Autodesk Fusion 360 part; units mm, degrees
(part 5 of 7)
  spline S10 degree 5 poles (-24.1252, -41.4832) (-24.1281, -41.4894) (-24.1337, -41.5019) (-24.1416, -41.5208) (-24.1514, -41.5463) (-24.1624, -41.5787) (-24.1725, -41.6115) (-24.1821, -41.6445) (-24.1913, -41.6776) (-24.2004, -41.7108) (-24.2093, -41.7442) (-24.2179, -41.7776) (-24.2261, -41.8112) (-24.2339, -41.8449) (-24.2413, -41.8788) (-24.2483, -41.9128) (-24.255, -41.947) (-24.2613, -41.9813) (-24.2675, -42.0157) (-24.2734, -42.0502) (-24.279, -42.0847) (-24.2844, -42.1193) (-24.2896, -42.1541) (-24.2944, -42.1889) (-24.299, -42.2238) (-24.3034, -42.2588) (-24.3075, -42.2939) (-24.3114, -42.3291) (-24.315, -42.3643) (-24.3185, -42.3996) (-24.3217, -42.435) (-24.3247, -42.4705) (-24.3275, -42.506) (-24.33, -42.5416) (-24.3324, -42.5773) (-24.3345, -42.613) (-24.3364, -42.6488) (-24.3382, -42.6847) (-24.3397, -42.7206) (-24.341, -42.7565) (-24.3421, -42.7926) (-24.343, -42.8287) (-24.3438, -42.8648) (-24.3443, -42.901) (-24.3446, -42.9372) (-24.3448, -42.9735) (-24.3447, -43.0099) (-24.3445, -43.0463) (-24.3441, -43.0828) (-24.3435, -43.1193) (-24.3427, -43.1558) (-24.3418, -43.1924) (-24.3406, -43.229) (-24.3393, -43.2657) (-24.3378, -43.3024) (-24.3361, -43.3392) (-24.3342, -43.376) (-24.3322, -43.4129) (-24.33, -43.4497) (-24.3276, -43.4867) (-24.325, -43.5236) (-24.3223, -43.5606) (-24.3194, -43.5977) (-24.3163, -43.6348) (-24.3131, -43.6719) (-24.3097, -43.709) (-24.3061, -43.7462) (-24.3024, -43.7834) (-24.2985, -43.8206) (-24.2944, -43.8579) (-24.2901, -43.8952) (-24.2866, -43.9251) (-24.2839, -43.9475) (-24.2821, -43.9625) (-24.2811, -43.9699) knots 0 0 0 0 0 0 0.01428571 0.02857143 0.04285714 0.05714286 0.07142857 0.08571429 0.1 0.11428571 0.12857143 0.14285714 0.15714286 0.17142857 0.18571429 0.2 0.21428571 0.22857143 0.24285714 0.25714286 0.27142857 0.28571429 0.3 0.31428571 0.32857143 0.34285714 0.35714286 0.37142857 0.38571429 0.4 0.41428571 0.42857143 0.44285714 0.45714286 0.47142857 0.48571429 0.5 0.51428571 0.52857143 0.54285714 0.55714286 0.57142857 0.58571429 0.6 0.61428571 0.62857143 0.64285714 0.65714286 0.67142857 0.68571429 0.7 0.71428571 0.72857143 0.74285714 0.75714286 0.77142857 0.78571429 0.8 0.81428571 0.82857143 0.84285714 0.85714286 0.87142857 0.88571429 0.9 0.91428571 0.92857143 0.94285714 0.95714286 0.97142857 0.98571429 1 1 1 1 1 1
  arc A22 (-24.2811, -43.9699) -> (-23.453, -44.284) centre (-17.3506, -26.9445) ccw
  spline S11 degree 5 poles (-23.453, -44.284) (-23.4474, -44.279) (-23.4361, -44.2691) (-23.4192, -44.2541) (-23.3967, -44.2341) (-23.3688, -44.2089) (-23.341, -44.1837) (-23.3134, -44.1585) (-23.2859, -44.1331) (-23.2586, -44.1076) (-23.2314, -44.0821) (-23.2044, -44.0565) (-23.1775, -44.0307) (-23.1508, -44.0049) (-23.1242, -43.9791) (-23.0978, -43.9531) (-23.0715, -43.927) (-23.0454, -43.9009) (-23.0194, -43.8747) (-22.9936, -43.8483) (-22.968, -43.8219) (-22.9425, -43.7954) (-22.9172, -43.7689) (-22.892, -43.7422) (-22.867, -43.7155) (-22.8422, -43.6886) (-22.8176, -43.6617) (-22.7931, -43.6347) (-22.7688, -43.6076) (-22.7446, -43.5804) (-22.7207, -43.5531) (-22.6969, -43.5258) (-22.6733, -43.4983) (-22.6499, -43.4708) (-22.6266, -43.4432) (-22.6036, -43.4155) (-22.5807, -43.3877) (-22.558, -43.3598) (-22.5355, -43.3318) (-22.5132, -43.3037) (-22.4912, -43.2756) (-22.4693, -43.2473) (-22.4476, -43.219) (-22.4261, -43.1905) (-22.4048, -43.162) (-22.3838, -43.1334) (-22.3629, -43.1047) (-22.3423, -43.0759) (-22.3219, -43.047) (-22.3017, -43.018) (-22.2817, -42.9889) (-22.262, -42.9597) (-22.2426, -42.9304) (-22.2234, -42.901) (-22.2045, -42.8715) (-22.1858, -42.8419) (-22.1673, -42.8122) (-22.1491, -42.7824) (-22.1312, -42.7525) (-22.1135, -42.7225) (-22.0961, -42.6924) (-22.0792, -42.6621) (-22.0627, -42.6316) (-22.0466, -42.6011) (-22.0308, -42.5703) (-22.0154, -42.5395) (-22.0001, -42.5086) (-21.9851, -42.4777) (-21.9704, -42.4466) (-21.9562, -42.4154) (-21.943, -42.3838) (-21.9333, -42.3583) (-21.9267, -42.3389) (-21.9227, -42.3258) (-21.9207, -42.3193) knots -1 -1 -1 -1 -1 -1 -0.98571429 -0.97142857 -0.95714286 -0.94285714 -0.92857143 -0.91428571 -0.9 -0.88571429 -0.87142857 -0.85714286 -0.84285714 -0.82857143 -0.81428571 -0.8 -0.78571429 -0.77142857 -0.75714286 -0.74285714 -0.72857143 -0.71428571 -0.7 -0.68571429 -0.67142857 -0.65714286 -0.64285714 -0.62857143 -0.61428571 -0.6 -0.58571429 -0.57142857 -0.55714286 -0.54285714 -0.52857143 -0.51428571 -0.5 -0.48571429 -0.47142857 -0.45714286 -0.44285714 -0.42857143 -0.41428571 -0.4 -0.38571429 -0.37142857 -0.35714286 -0.34285714 -0.32857143 -0.31428571 -0.3 -0.28571429 -0.27142857 -0.25714286 -0.24285714 -0.22857143 -0.21428571 -0.2 -0.18571429 -0.17142857 -0.15714286 -0.14285714 -0.12857143 -0.11428571 -0.1 -0.08571429 -0.07142857 -0.05714286 -0.04285714 -0.02857143 -0.01428571 0 0 0 0 0 0
  line L11 (-21.9207, -42.3193) -> (-21.8906, -42.2182)
  arc A23 (-21.2841, -41.8777) -> (-21.8906, -42.2182) centre (-21.4115, -42.3612) ccw
  arc A24 (-21.2841, -41.8777) -> (-20.8075, -41.9952) centre (-17.3506, -26.9445) ccw
  arc A25 (-20.4288, -42.5785) -> (-20.8075, -41.9952) centre (-20.9195, -42.4825) ccw
  line L12 (-20.4288, -42.5785) -> (-20.449, -42.682)
  spline S12 degree 5 poles (-20.449, -42.682) (-20.4503, -42.6887) (-20.4528, -42.7022) (-20.456, -42.7224) (-20.4593, -42.7495) (-20.4622, -42.7836) (-20.4642, -42.8179) (-20.4656, -42.8522) (-20.4667, -42.8866) (-20.4675, -42.921) (-20.4682, -42.9555) (-20.4685, -42.99) (-20.4685, -43.0246) (-20.468, -43.0592) (-20.4671, -43.0939) (-20.4657, -43.1286) (-20.464, -43.1634) (-20.462, -43.1982) (-20.4597, -43.2331) (-20.4572, -43.2679) (-20.4544, -43.3028) (-20.4513, -43.3378) (-20.448, -43.3727) (-20.4444, -43.4077) (-20.4406, -43.4427) (-20.4364, -43.4777) (-20.432, -43.5128) (-20.4273, -43.5479) (-20.4225, -43.583) (-20.4173, -43.6181) (-20.412, -43.6532) (-20.4064, -43.6883) (-20.4006, -43.7235) (-20.3946, -43.7587) (-20.3883, -43.7939) (-20.3819, -43.8291) (-20.3752, -43.8643) (-20.3682, -43.8995) (-20.3611, -43.9347) (-20.3538, -43.97) (-20.3463, -44.0052) (-20.3385, -44.0405) (-20.3306, -44.0758) (-20.3224, -44.111) (-20.3141, -44.1463) (-20.3055, -44.1816) (-20.2968, -44.2169) (-20.2879, -44.2522) (-20.2787, -44.2875) (-20.2694, -44.3228) (-20.2599, -44.358) (-20.2502, -44.3933) (-20.2404, -44.4286) (-20.2303, -44.4639) (-20.22, -44.4992) (-20.2096, -44.5345) (-20.199, -44.5698) (-20.1882, -44.6051) (-20.1772, -44.6404) (-20.1661, -44.6757) (-20.1547, -44.711) (-20.1432, -44.7462) (-20.1315, -44.7815) (-20.1197, -44.8168) (-20.1077, -44.852) (-20.0955, -44.8873) (-20.0831, -44.9225) (-20.0705, -44.9578) (-20.0578, -44.993) (-20.045, -45.0282) (-20.0319, -45.0634) (-20.0213, -45.0916) (-20.0133, -45.1127) (-20.008, -45.1268) (-20.0053, -45.1338) knots 0 0 0 0 0 0 0.01428571 0.02857143 0.04285714 0.05714286 0.07142857 0.08571429 0.1 0.11428571 0.12857143 0.14285714 0.15714286 0.17142857 0.18571429 0.2 0.21428571 0.22857143 0.24285714 0.25714286 0.27142857 0.28571429 0.3 0.31428571 0.32857143 0.34285714 0.35714286 0.37142857 0.38571429 0.4 0.41428571 0.42857143 0.44285714 0.45714286 0.47142857 0.48571429 0.5 0.51428571 0.52857143 0.54285714 0.55714286 0.57142857 0.58571429 0.6 0.61428571 0.62857143 0.64285714 0.65714286 0.67142857 0.68571429 0.7 0.71428571 0.72857143 0.74285714 0.75714286 0.77142857 0.78571429 0.8 0.81428571 0.82857143 0.84285714 0.85714286 0.87142857 0.88571429 0.9 0.91428571 0.92857143 0.94285714 0.95714286 0.97142857 0.98571429 1 1 1 1 1 1
  arc A26 (-20.0053, -45.1338) -> (-19.1261, -45.2405) centre (-17.3506, -26.9445) ccw
  spline S13 degree 5 poles (-19.1261, -45.2405) (-19.1218, -45.2344) (-19.1132, -45.222) (-19.1004, -45.2034) (-19.0834, -45.1786) (-19.0623, -45.1475) (-19.0414, -45.1164) (-19.0206, -45.0852) (-19, -45.054) (-18.9795, -45.0228) (-18.9592, -44.9915) (-18.9391, -44.9601) (-18.9192, -44.9287) (-18.8994, -44.8973) (-18.8798, -44.8658) (-18.8603, -44.8342) (-18.8411, -44.8026) (-18.822, -44.771) (-18.803, -44.7393) (-18.7843, -44.7076) (-18.7657, -44.6758) (-18.7473, -44.644) (-18.7291, -44.6121) (-18.711, -44.5802) (-18.6932, -44.5483) (-18.6755, -44.5163) (-18.658, -44.4843) (-18.6407, -44.4522) (-18.6236, -44.42) (-18.6067, -44.3879) (-18.5899, -44.3557) (-18.5734, -44.3234) (-18.557, -44.2911) (-18.5409, -44.2588) (-18.5249, -44.2264) (-18.5092, -44.194) (-18.4936, -44.1615) (-18.4783, -44.129) (-18.4631, -44.0964) (-18.4482, -44.0639) (-18.4335, -44.0312) (-18.419, -43.9986) (-18.4047, -43.9658) (-18.3907, -43.9331) (-18.3769, -43.9003) (-18.3633, -43.8675) (-18.3499, -43.8346) (-18.3367, -43.8017) (-18.3238, -43.7688) (-18.3112, -43.7358) (-18.2988, -43.7028) (-18.2866, -43.6697) (-18.2747, -43.6366) (-18.2632, -43.6034) (-18.2518, -43.5703) (-18.2408, -43.537) (-18.23, -43.5038) (-18.2194, -43.4705) (-18.2091, -43.4372) (-18.1992, -43.4038) (-18.1895, -43.3704) (-18.1803, -43.337) (-18.1716, -43.3035) (-18.1633, -43.2699) (-18.1553, -43.2363) (-18.1477, -43.2027) (-18.1403, -43.1691) (-18.1331, -43.1354) (-18.1262, -43.1017) (-18.12, -43.068) (-18.1146, -43.0342) (-18.1114, -43.0071) (-18.1097, -42.9867) (-18.1088, -42.973) (-18.1085, -42.9662) knots -1 -1 -1 -1 -1 -1 -0.98571429 -0.97142857 -0.95714286 -0.94285714 -0.92857143 -0.91428571 -0.9 -0.88571429 -0.87142857 -0.85714286 -0.84285714 -0.82857143 -0.81428571 -0.8 -0.78571429 -0.77142857 -0.75714286 -0.74285714 -0.72857143 -0.71428571 -0.7 -0.68571429 -0.67142857 -0.65714286 -0.64285714 -0.62857143 -0.61428571 -0.6 -0.58571429 -0.57142857 -0.55714286 -0.54285714 -0.52857143 -0.51428571 -0.5 -0.48571429 -0.47142857 -0.45714286 -0.44285714 -0.42857143 -0.41428571 -0.4 -0.38571429 -0.37142857 -0.35714286 -0.34285714 -0.32857143 -0.31428571 -0.3 -0.28571429 -0.27142857 -0.25714286 -0.24285714 -0.22857143 -0.21428571 -0.2 -0.18571429 -0.17142857 -0.15714286 -0.14285714 -0.12857143 -0.11428571 -0.1 -0.08571429 -0.07142857 -0.05714286 -0.04285714 -0.02857143 -0.01428571 0 0 0 0 0 0
  line L13 (-18.1085, -42.9662) -> (-18.1034, -42.8608)
  arc A27 (-17.596, -42.3851) -> (-18.1034, -42.8608) centre (-17.604, -42.8851) ccw
  arc A28 (-17.596, -42.3851) -> (-17.1052, -42.3851) centre (-17.3506, -26.9445) ccw
  arc A29 (-16.5978, -42.8608) -> (-17.1052, -42.3851) centre (-17.0973, -42.8851) ccw
  line L14 (-16.5978, -42.8608) -> (-16.5927, -42.9662)
  spline S14 degree 5 poles (-16.5927, -42.9662) (-16.5924, -42.973) (-16.5916, -42.9867) (-16.5898, -43.0071) (-16.5866, -43.0342) (-16.5813, -43.068) (-16.575, -43.1017) (-16.5681, -43.1354) (-16.5609, -43.1691) (-16.5535, -43.2027) (-16.5459, -43.2363) (-16.538, -43.2699) (-16.5297, -43.3035) (-16.5209, -43.337) (-16.5117, -43.3704) (-16.5021, -43.4038) (-16.4921, -43.4372) (-16.4818, -43.4705) (-16.4712, -43.5038) (-16.4604, -43.537) (-16.4494, -43.5703) (-16.4381, -43.6034) (-16.4265, -43.6366) (-16.4146, -43.6697) (-16.4025, -43.7028) (-16.3901, -43.7358) (-16.3774, -43.7688) (-16.3645, -43.8017) (-16.3513, -43.8346) (-16.338, -43.8675) (-16.3244, -43.9003) (-16.3106, -43.9331) (-16.2965, -43.9658) (-16.2822, -43.9986) (-16.2677, -44.0312) (-16.253, -44.0639) (-16.2381, -44.0964) (-16.223, -44.129) (-16.2076, -44.1615) (-16.1921, -44.194) (-16.1763, -44.2264) (-16.1604, -44.2588) (-16.1442, -44.2911) (-16.1279, -44.3234) (-16.1113, -44.3557) (-16.0946, -44.3879) (-16.0776, -44.42) (-16.0605, -44.4522) (-16.0432, -44.4843) (-16.0257, -44.5163) (-16.008, -44.5483) (-15.9902, -44.5802) (-15.9721, -44.6121) (-15.9539, -44.644) (-15.9355, -44.6758) (-15.9169, -44.7076) (-15.8982, -44.7393) (-15.8793, -44.771) (-15.8602, -44.8026) (-15.8409, -44.8342) (-15.8215, -44.8658) (-15.8018, -44.8973) (-15.7821, -44.9287) (-15.7621, -44.9601) (-15.742, -44.9915) (-15.7217, -45.0228) (-15.7013, -45.054) (-15.6807, -45.0852) (-15.6599, -45.1164) (-15.639, -45.1475) (-15.6179, -45.1786) (-15.6009, -45.2034) (-15.588, -45.222) (-15.5795, -45.2344) (-15.5752, -45.2405) knots 0 0 0 0 0 0 0.01428571 0.02857143 0.04285714 0.05714286 0.07142857 0.08571429 0.1 0.11428571 0.12857143 0.14285714 0.15714286 0.17142857 0.18571429 0.2 0.21428571 0.22857143 0.24285714 0.25714286 0.27142857 0.28571429 0.3 0.31428571 0.32857143 0.34285714 0.35714286 0.37142857 0.38571429 0.4 0.41428571 0.42857143 0.44285714 0.45714286 0.47142857 0.48571429 0.5 0.51428571 0.52857143 0.54285714 0.55714286 0.57142857 0.58571429 0.6 0.61428571 0.62857143 0.64285714 0.65714286 0.67142857 0.68571429 0.7 0.71428571 0.72857143 0.74285714 0.75714286 0.77142857 0.78571429 0.8 0.81428571 0.82857143 0.84285714 0.85714286 0.87142857 0.88571429 0.9 0.91428571 0.92857143 0.94285714 0.95714286 0.97142857 0.98571429 1 1 1 1 1 1
  arc A30 (-15.5752, -45.2405) -> (-14.696, -45.1338) centre (-17.3506, -26.9445) ccw
  spline S15 degree 5 poles (-14.696, -45.1338) (-14.6933, -45.1268) (-14.6879, -45.1127) (-14.6799, -45.0916) (-14.6693, -45.0634) (-14.6563, -45.0282) (-14.6434, -44.993) (-14.6307, -44.9578) (-14.6182, -44.9225) (-14.6058, -44.8873) (-14.5936, -44.852) (-14.5816, -44.8168) (-14.5697, -44.7815) (-14.558, -44.7462) (-14.5465, -44.711) (-14.5352, -44.6757) (-14.524, -44.6404) (-14.513, -44.6051) (-14.5023, -44.5698) (-14.4916, -44.5345) (-14.4812, -44.4992) (-14.471, -44.4639) (-14.4609, -44.4286) (-14.451, -44.3933) (-14.4413, -44.358) (-14.4318, -44.3228) (-14.4225, -44.2875) (-14.4134, -44.2522) (-14.4044, -44.2169) (-14.3957, -44.1816) (-14.3871, -44.1463) (-14.3788, -44.111) (-14.3707, -44.0758) (-14.3627, -44.0405) (-14.355, -44.0052) (-14.3474, -43.97) (-14.3401, -43.9347) (-14.333, -43.8995) (-14.3261, -43.8643) (-14.3194, -43.8291) (-14.3129, -43.7939) (-14.3067, -43.7587) (-14.3006, -43.7235) (-14.2948, -43.6883) (-14.2892, -43.6532) (-14.2839, -43.6181) (-14.2788, -43.583) (-14.2739, -43.5479) (-14.2692, -43.5128) (-14.2648, -43.4777) (-14.2607, -43.4427) (-14.2568, -43.4077) (-14.2532, -43.3727) (-14.2499, -43.3378) (-14.2469, -43.3028) (-14.2441, -43.2679) (-14.2415, -43.2331) (-14.2393, -43.1982) (-14.2372, -43.1634) (-14.2355, -43.1286) (-14.2342, -43.0939) (-14.2332, -43.0592) (-14.2328, -43.0246) (-14.2327, -42.99) (-14.2331, -42.9555) (-14.2337, -42.921) (-14.2346, -42.8866) (-14.2356, -42.8522) (-14.237, -42.8179) (-14.239, -42.7836) (-14.2419, -42.7495) (-14.2453, -42.7224) (-14.2485, -42.7022) (-14.2509, -42.6887) (-14.2522, -42.682) knots -1 -1 -1 -1 -1 -1 -0.98571429 -0.97142857 -0.95714286 -0.94285714 -0.92857143 -0.91428571 -0.9 -0.88571429 -0.87142857 -0.85714286 -0.84285714 -0.82857143 -0.81428571 -0.8 -0.78571429 -0.77142857 -0.75714286 -0.74285714 -0.72857143 -0.71428571 -0.7 -0.68571429 -0.67142857 -0.65714286 -0.64285714 -0.62857143 -0.61428571 -0.6 -0.58571429 -0.57142857 -0.55714286 -0.54285714 -0.52857143 -0.51428571 -0.5 -0.48571429 -0.47142857 -0.45714286 -0.44285714 -0.42857143 -0.41428571 -0.4 -0.38571429 -0.37142857 -0.35714286 -0.34285714 -0.32857143 -0.31428571 -0.3 -0.28571429 -0.27142857 -0.25714286 -0.24285714 -0.22857143 -0.21428571 -0.2 -0.18571429 -0.17142857 -0.15714286 -0.14285714 -0.12857143 -0.11428571 -0.1 -0.08571429 -0.07142857 -0.05714286 -0.04285714 -0.02857143 -0.01428571 0 0 0 0 0 0
  line L15 (-14.2522, -42.682) -> (-14.2725, -42.5785)
  arc A31 (-13.8937, -41.9952) -> (-14.2725, -42.5785) centre (-13.7818, -42.4825) ccw
  arc A32 (-13.8937, -41.9952) -> (-13.4171, -41.8777) centre (-17.3506, -26.9445) ccw
  arc A33 (-12.8107, -42.2182) -> (-13.4171, -41.8777) centre (-13.2898, -42.3612) ccw
  line L16 (-12.8107, -42.2182) -> (-12.7805, -42.3193)
  spline S16 degree 5 poles (-12.7805, -42.3193) (-12.7786, -42.3258) (-12.7745, -42.3389) (-12.7679, -42.3583) (-12.7583, -42.3838) (-12.745, -42.4154) (-12.7308, -42.4466) (-12.7161, -42.4777) (-12.7011, -42.5086) (-12.6858, -42.5395) (-12.6704, -42.5703) (-12.6547, -42.6011) (-12.6386, -42.6316) (-12.622, -42.6621) (-12.6051, -42.6924) (-12.5878, -42.7225) (-12.5701, -42.7525) (-12.5521, -42.7824) (-12.5339, -42.8122) (-12.5155, -42.8419) (-12.4968, -42.8715) (-12.4778, -42.901) (-12.4587, -42.9304) (-12.4392, -42.9597) (-12.4195, -42.9889) (-12.3996, -43.018) (-12.3794, -43.047) (-12.359, -43.0759) (-12.3383, -43.1047) (-12.3175, -43.1334) (-12.2964, -43.162) (-12.2751, -43.1905) (-12.2537, -43.219) (-12.232, -43.2473) (-12.2101, -43.2756) (-12.188, -43.3037) (-12.1657, -43.3318) (-12.1432, -43.3598) (-12.1205, -43.3877) (-12.0977, -43.4155) (-12.0746, -43.4432) (-12.0514, -43.4708) (-12.0279, -43.4983) (-12.0043, -43.5258) (-11.9806, -43.5531) (-11.9566, -43.5804) (-11.9325, -43.6076) (-11.9082, -43.6347) (-11.8837, -43.6617) (-11.859, -43.6886) (-11.8342, -43.7155) (-11.8092, -43.7422) (-11.7841, -43.7689) (-11.7587, -43.7954) (-11.7333, -43.8219) (-11.7076, -43.8483) (-11.6818, -43.8747) (-11.6559, -43.9009) (-11.6297, -43.927) (-11.6035, -43.9531) (-11.577, -43.9791) (-11.5505, -44.0049) (-11.5237, -44.0307) (-11.4968, -44.0565) (-11.4698, -44.0821) (-11.4426, -44.1076) (-11.4153, -44.1331) (-11.3878, -44.1585) (-11.3602, -44.1837) (-11.3324, -44.2089) (-11.3045, -44.2341) (-11.2821, -44.2541) (-11.2652, -44.2691) (-11.2539, -44.279) (-11.2482, -44.284) knots 0 0 0 0 0 0 0.01428571 0.02857143 0.04285714 0.05714286 0.07142857 0.08571429 0.1 0.11428571 0.12857143 0.14285714 0.15714286 0.17142857 0.18571429 0.2 0.21428571 0.22857143 0.24285714 0.25714286 0.27142857 0.28571429 0.3 0.31428571 0.32857143 0.34285714 0.35714286 0.37142857 0.38571429 0.4 0.41428571 0.42857143 0.44285714 0.45714286 0.47142857 0.48571429 0.5 0.51428571 0.52857143 0.54285714 0.55714286 0.57142857 0.58571429 0.6 0.61428571 0.62857143 0.64285714 0.65714286 0.67142857 0.68571429 0.7 0.71428571 0.72857143 0.74285714 0.75714286 0.77142857 0.78571429 0.8 0.81428571 0.82857143 0.84285714 0.85714286 0.87142857 0.88571429 0.9 0.91428571 0.92857143 0.94285714 0.95714286 0.97142857 0.98571429 1 1 1 1 1 1
  arc A34 (-11.2482, -44.284) -> (-10.4201, -43.9699) centre (-17.3506, -26.9445) ccw
  spline S17 degree 5 poles (-10.4201, -43.9699) (-10.4192, -43.9625) (-10.4173, -43.9475) (-10.4146, -43.9251) (-10.4111, -43.8952) (-10.4069, -43.8579) (-10.4028, -43.8206) (-10.3989, -43.7834) (-10.3951, -43.7462) (-10.3915, -43.709) (-10.3881, -43.6719) (-10.3849, -43.6348) (-10.3818, -43.5977) (-10.3789, -43.5606) (-10.3762, -43.5236) (-10.3736, -43.4867) (-10.3713, -43.4497) (-10.369, -43.4129) (-10.367, -43.376) (-10.3651, -43.3392) (-10.3635, -43.3024) (-10.362, -43.2657) (-10.3606, -43.229) (-10.3595, -43.1924) (-10.3585, -43.1558) (-10.3577, -43.1193) (-10.3571, -43.0828) (-10.3567, -43.0463) (-10.3565, -43.0099) (-10.3564, -42.9735) (-10.3566, -42.9372) (-10.3569, -42.901) (-10.3575, -42.8648) (-10.3582, -42.8287) (-10.3591, -42.7926) (-10.3602, -42.7565) (-10.3616, -42.7206) (-10.3631, -42.6847) (-10.3648, -42.6488) (-10.3667, -42.613) (-10.3689, -42.5773) (-10.3712, -42.5416) (-10.3738, -42.506) (-10.3765, -42.4705) (-10.3795, -42.435) (-10.3828, -42.3996) (-10.3862, -42.3643) (-10.3899, -42.3291) (-10.3937, -42.2939) (-10.3978, -42.2588) (-10.4022, -42.2238) (-10.4068, -42.1889) (-10.4117, -42.1541) (-10.4168, -42.1193) (-10.4222, -42.0847) (-10.4279, -42.0502) (-10.4338, -42.0157) (-10.4399, -41.9813) (-10.4463, -41.947) (-10.4529, -41.9128) (-10.4599, -41.8788) (-10.4673, -41.8449) (-10.4751, -41.8112) (-10.4834, -41.7776) (-10.492, -41.7442) (-10.5008, -41.7108) (-10.5099, -41.6776) (-10.5192, -41.6445) (-10.5288, -41.6115) (-10.5389, -41.5787) (-10.5498, -41.5463) (-10.5596, -41.5208) (-10.5675, -41.5019) (-10.5732, -41.4894) (-10.576, -41.4832) knots -1 -1 -1 -1 -1 -1 -0.98571429 -0.97142857 -0.95714286 -0.94285714 -0.92857143 -0.91428571 -0.9 -0.88571429 -0.87142857 -0.85714286 -0.84285714 -0.82857143 -0.81428571 -0.8 -0.78571429 -0.77142857 -0.75714286 -0.74285714 -0.72857143 -0.71428571 -0.7 -0.68571429 -0.67142857 -0.65714286 -0.64285714 -0.62857143 -0.61428571 -0.6 -0.58571429 -0.57142857 -0.55714286 -0.54285714 -0.52857143 -0.51428571 -0.5 -0.48571429 -0.47142857 -0.45714286 -0.44285714 -0.42857143 -0.41428571 -0.4 -0.38571429 -0.37142857 -0.35714286 -0.34285714 -0.32857143 -0.31428571 -0.3 -0.28571429 -0.27142857 -0.25714286 -0.24285714 -0.22857143 -0.21428571 -0.2 -0.18571429 -0.17142857 -0.15714286 -0.14285714 -0.12857143 -0.11428571 -0.1 -0.08571429 -0.07142857 -0.05714286 -0.04285714 -0.02857143 -0.01428571 0 0 0 0 0 0
  line L17 (-10.576, -41.4832) -> (-10.6205, -41.3876)
  arc A35 (-10.3923, -40.7306) -> (-10.6205, -41.3876) centre (-10.167, -41.1769) ccw
  arc A36 (-10.3923, -40.7306) -> (-9.9577, -40.5025) centre (-17.3506, -26.9445) ccw
  arc A37 (-9.2874, -40.6879) -> (-9.9577, -40.5025) centre (-9.7183, -40.9414) ccw
  line L18 (-9.2874, -40.6879) -> (-9.2339, -40.7788)
  spline S18 degree 5 poles (-9.2339, -40.7788) (-9.2304, -40.7847) (-9.2233, -40.7964) (-9.2123, -40.8137) (-9.1968, -40.8362) (-9.1764, -40.8636) (-9.1552, -40.8906) (-9.1335, -40.9172) (-9.1115, -40.9437) (-9.0893, -40.97) (-9.0669, -40.9962) (-9.0443, -41.0223) (-9.0213, -41.0481) (-8.998, -41.0737) (-8.9743, -41.0991) (-8.9502, -41.1242) (-8.9259, -41.1491) (-8.9013, -41.1738) (-8.8765, -41.1984) (-8.8515, -41.2228) (-8.8262, -41.2471) (-8.8008, -41.2712) (-8.7751, -41.2951) (-8.7493, -41.3189) (-8.7231, -41.3426) (-8.6968, -41.366) (-8.6703, -41.3894) (-8.6435, -41.4125) (-8.6166, -41.4356) (-8.5895, -41.4585) (-8.5622, -41.4812) (-8.5347, -41.5038) (-8.507, -41.5263) (-8.4792, -41.5486) (-8.4512, -41.5708) (-8.423, -41.5929) (-8.3946, -41.6148) (-8.3661, -41.6366) (-8.3374, -41.6582) (-8.3085, -41.6797) (-8.2795, -41.7011) (-8.2504, -41.7224) (-8.221, -41.7435) (-8.1915, -41.7645) (-8.1619, -41.7854) (-8.1321, -41.8061) (-8.1022, -41.8267) (-8.0721, -41.8472) (-8.0418, -41.8676) (-8.0115, -41.8878) (-7.9809, -41.908) (-7.9503, -41.9279) (-7.9195, -41.9478) (-7.8885, -41.9676) (-7.8575, -41.9872) (-7.8262, -42.0067) (-7.7949, -42.0261) (-7.7634, -42.0453) (-7.7318, -42.0645) (-7.7, -42.0835) (-7.6682, -42.1024) (-7.6362, -42.1211) (-7.604, -42.1398) (-7.5718, -42.1583) (-7.5394, -42.1767) (-7.5069, -42.195) (-7.4743, -42.2132) (-7.4415, -42.2313) (-7.4086, -42.2492) (-7.3756, -42.267) (-7.3425, -42.2847) (-7.3159, -42.2988) (-7.296, -42.3093) (-7.2826, -42.3163) (-7.2759, -42.3197) knots 0 0 0 0 0 0 0.01428571 0.02857143 0.04285714 0.05714286 0.07142857 0.08571429 0.1 0.11428571 0.12857143 0.14285714 0.15714286 0.17142857 0.18571429 0.2 0.21428571 0.22857143 0.24285714 0.25714286 0.27142857 0.28571429 0.3 0.31428571 0.32857143 0.34285714 0.35714286 0.37142857 0.38571429 0.4 0.41428571 0.42857143 0.44285714 0.45714286 0.47142857 0.48571429 0.5 0.51428571 0.52857143 0.54285714 0.55714286 0.57142857 0.58571429 0.6 0.61428571 0.62857143 0.64285714 0.65714286 0.67142857 0.68571429 0.7 0.71428571 0.72857143 0.74285714 0.75714286 0.77142857 0.78571429 0.8 0.81428571 0.82857143 0.84285714 0.85714286 0.87142857 0.88571429 0.9 0.91428571 0.92857143 0.94285714 0.95714286 0.97142857 0.98571429 1 1 1 1 1 1
  arc A38 (-7.2759, -42.3197) -> (-6.547, -41.8166) centre (-17.3506, -26.9445) ccw
  spline S19 degree 5 poles (-6.547, -41.8166) (-6.5479, -41.8092) (-6.5497, -41.7942) (-6.5524, -41.7718) (-6.5562, -41.7419) (-6.561, -41.7047) (-6.5659, -41.6675) (-6.5711, -41.6304) (-6.5763, -41.5934) (-6.5818, -41.5565) (-6.5873, -41.5196) (-6.5931, -41.4828) (-6.599, -41.446) (-6.605, -41.4094) (-6.6112, -41.3728) (-6.6176, -41.3363) (-6.6241, -41.2999) (-6.6308, -41.2635) (-6.6376, -41.2272) (-6.6446, -41.1911) (-6.6518, -41.155) (-6.6591, -41.1189) (-6.6666, -41.083) (-6.6743, -41.0472) (-6.6821, -41.0114) (-6.6901, -40.9757) (-6.6982, -40.9402) (-6.7065, -40.9047) (-6.715, -40.8693) (-6.7237, -40.834) (-6.7325, -40.7987) (-6.7415, -40.7636) (-6.7507, -40.7286) (-6.7601, -40.6937) (-6.7696, -40.6589) (-6.7793, -40.6242) (-6.7892, -40.5896) (-6.7993, -40.555) (-6.8095, -40.5206) (-6.8199, -40.4864) (-6.8306, -40.4522) (-6.8414, -40.4181) (-6.8524, -40.3842) (-6.8636, -40.3503) (-6.875, -40.3166) (-6.8866, -40.283) (-6.8984, -40.2496) (-6.9103, -40.2162) (-6.9225, -40.183) (-6.9349, -40.1499) (-6.9475, -40.117) (-6.9604, -40.0842) (-6.9734, -40.0515) (-6.9867, -40.019) (-7.0003, -39.9867) (-7.014, -39.9545) (-7.028, -39.9224) (-7.0422, -39.8905) (-7.0565, -39.8588) (-7.0712, -39.8272) (-7.0861, -39.7958) (-7.1014, -39.7646) (-7.1171, -39.7338) (-7.1331, -39.7031) (-7.1495, -39.6727) (-7.1661, -39.6425) (-7.1828, -39.6124) (-7.1997, -39.5825) (-7.2169, -39.5527) (-7.2346, -39.5233) (-7.253, -39.4945) (-7.2686, -39.472) (-7.2808, -39.4556) (-7.2893, -39.4448) (-7.2936, -39.4395) knots -1 -1 -1 -1 -1 -1 -0.98571429 -0.97142857 -0.95714286 -0.94285714 -0.92857143 -0.91428571 -0.9 -0.88571429 -0.87142857 -0.85714286 -0.84285714 -0.82857143 -0.81428571 -0.8 -0.78571429 -0.77142857 -0.75714286 -0.74285714 -0.72857143 -0.71428571 -0.7 -0.68571429 -0.67142857 -0.65714286 -0.64285714 -0.62857143 -0.61428571 -0.6 -0.58571429 -0.57142857 -0.55714286 -0.54285714 -0.52857143 -0.51428571 -0.5 -0.48571429 -0.47142857 -0.45714286 -0.44285714 -0.42857143 -0.41428571 -0.4 -0.38571429 -0.37142857 -0.35714286 -0.34285714 -0.32857143 -0.31428571 -0.3 -0.28571429 -0.27142857 -0.25714286 -0.24285714 -0.22857143 -0.21428571 -0.2 -0.18571429 -0.17142857 -0.15714286 -0.14285714 -0.12857143 -0.11428571 -0.1 -0.08571429 -0.07142857 -0.05714286 -0.04285714 -0.02857143 -0.01428571 0 0 0 0 0 0
  line L19 (-7.2936, -39.4395) -> (-7.3596, -39.3572)
  arc A39 (-7.2953, -38.6647) -> (-7.3596, -39.3572) centre (-6.9697, -39.0442) ccw
  arc A40 (-7.2953, -38.6647) -> (-6.9279, -38.3392) centre (-17.3506, -26.9445) ccw
  arc A41 (-6.2327, -38.3589) -> (-6.9279, -38.3392) centre (-6.5904, -38.7082) ccw
  line L20 (-6.2327, -38.3589) -> (-6.159, -38.4343)
  spline S20 degree 5 poles (-6.159, -38.4343) (-6.1542, -38.4392) (-6.1445, -38.4489) (-6.1297, -38.463) (-6.1093, -38.4812) (-6.0829, -38.503) (-6.0558, -38.524) (-6.0283, -38.5447) (-6.0007, -38.5651) (-5.9728, -38.5854) (-5.9448, -38.6055) (-5.9166, -38.6254) (-5.8881, -38.645) (-5.8593, -38.6642) (-5.8303, -38.6832) (-5.8009, -38.7018) (-5.7713, -38.7201) (-5.7415, -38.7383) (-5.7116, -38.7562) (-5.6814, -38.7739) (-5.6511, -38.7914) (-5.6206, -38.8088) (-5.59, -38.8259) (-5.5592, -38.8428) (-5.5281, -38.8595) (-5.497, -38.876) (-5.4656, -38.8923) (-5.4341, -38.9084) (-5.4024, -38.9243) (-5.3706, -38.94) (-5.3387, -38.9556) (-5.3066, -38.971) (-5.2744, -38.9862) (-5.242, -39.0012) (-5.2095, -39.016) (-5.1768, -39.0307) (-5.144, -39.0452) (-5.1111, -39.0595) (-5.0781, -39.0736) (-5.0449, -39.0876) (-5.0116, -39.1015) (-4.9782, -39.1151) (-4.9447, -39.1286) (-4.911, -39.142) (-4.8772, -39.1551) (-4.8434, -39.1681) (-4.8093, -39.181) (-4.7752, -39.1937) (-4.741, -39.2062) (-4.7067, -39.2186) (-4.6722, -39.2308) (-4.6377, -39.2429) (-4.603, -39.2548) (-4.5682, -39.2666) (-4.5334, -39.2782) (-4.4984, -39.2897) (-4.4633, -39.301) (-4.4281, -39.3121) (-4.3929, -39.3232) (-4.3575, -39.334) (-4.322, -39.3447) (-4.2864, -39.3553) (-4.2508, -39.3657) (-4.215, -39.376) (-4.1792, -39.3861) (-4.1432, -39.3961) (-4.1072, -39.406) (-4.0711, -39.4156) (-4.0349, -39.4252) (-3.9986, -39.4346) (-3.9622, -39.4439) (-3.933, -39.4512) (-3.9111, -39.4566) (-3.8965, -39.4602) (-3.8891, -39.4619) knots 0 0 0 0 0 0 0.01428571 0.02857143 0.04285714 0.05714286 0.07142857 0.08571429 0.1 0.11428571 0.12857143 0.14285714 0.15714286 0.17142857 0.18571429 0.2 0.21428571 0.22857143 0.24285714 0.25714286 0.27142857 0.28571429 0.3 0.31428571 0.32857143 0.34285714 0.35714286 0.37142857 0.38571429 0.4 0.41428571 0.42857143 0.44285714 0.45714286 0.47142857 0.48571429 0.5 0.51428571 0.52857143 0.54285714 0.55714286 0.57142857 0.58571429 0.6 0.61428571 0.62857143 0.64285714 0.65714286 0.67142857 0.68571429 0.7 0.71428571 0.72857143 0.74285714 0.75714286 0.77142857 0.78571429 0.8 0.81428571 0.82857143 0.84285714 0.85714286 0.87142857 0.88571429 0.9 0.91428571 0.92857143 0.94285714 0.95714286 0.97142857 0.98571429 1 1 1 1 1 1
  arc A42 (-3.8891, -39.4619) -> (-3.3018, -38.799) centre (-17.3506, -26.9445) ccw
  spline S21 degree 5 poles (-3.3018, -38.799) (-3.3045, -38.792) (-3.3098, -38.7779) (-3.3178, -38.7568) (-3.3286, -38.7287) (-3.3422, -38.6937) (-3.3559, -38.6588) (-3.3697, -38.624) (-3.3837, -38.5893) (-3.3978, -38.5547) (-3.412, -38.5202) (-3.4264, -38.4859) (-3.4409, -38.4516) (-3.4556, -38.4175) (-3.4704, -38.3834) (-3.4853, -38.3495) (-3.5003, -38.3157) (-3.5155, -38.282) (-3.5308, -38.2484) (-3.5463, -38.215) (-3.5619, -38.1816) (-3.5776, -38.1484) (-3.5935, -38.1153) (-3.6095, -38.0823) (-3.6256, -38.0495) (-3.6419, -38.0168) (-3.6584, -37.9842) (-3.6749, -37.9517) (-3.6917, -37.9194) (-3.7085, -37.8872) (-3.7255, -37.8551) (-3.7427, -37.8232) (-3.76, -37.7913) (-3.7774, -37.7597) (-3.795, -37.7282) (-3.8127, -37.6968) (-3.8306, -37.6655) (-3.8486, -37.6344) (-3.8668, -37.6035) (-3.8852, -37.5727) (-3.9037, -37.5421) (-3.9223, -37.5116) (-3.9411, -37.4812) (-3.9601, -37.4511) (-3.9792, -37.4211) (-3.9985, -37.3912) (-4.018, -37.3616) (-4.0376, -37.332) (-4.0574, -37.3027) (-4.0773, -37.2735) (-4.0974, -37.2446) (-4.1177, -37.2158) (-4.1383, -37.1872) (-4.1589, -37.1589) (-4.1798, -37.1307) (-4.2009, -37.1027) (-4.2221, -37.075) (-4.2435, -37.0474) (-4.2651, -37.02) (-4.2869, -36.9928) (-4.3089, -36.9659) (-4.3312, -36.9393) (-4.3538, -36.9131) (-4.3767, -36.8872) (-4.3998, -36.8616) (-4.4232, -36.8362) (-4.4466, -36.811) (-4.4703, -36.786) (-4.4941, -36.7612) (-4.5182, -36.7369) (-4.543, -36.7133) (-4.5635, -36.6952) (-4.5794, -36.6822) (-4.5901, -36.6737) (-4.5955, -36.6696) knots -1 -1 -1 -1 -1 -1 -0.98571429 -0.97142857 -0.95714286 -0.94285714 -0.92857143 -0.91428571 -0.9 -0.88571429 -0.87142857 -0.85714286 -0.84285714 -0.82857143 -0.81428571 -0.8 -0.78571429 -0.77142857 -0.75714286 -0.74285714 -0.72857143 -0.71428571 -0.7 -0.68571429 -0.67142857 -0.65714286 -0.64285714 -0.62857143 -0.61428571 -0.6 -0.58571429 -0.57142857 -0.55714286 -0.54285714 -0.52857143 -0.51428571 -0.5 -0.48571429 -0.47142857 -0.45714286 -0.44285714 -0.42857143 -0.41428571 -0.4 -0.38571429 -0.37142857 -0.35714286 -0.34285714 -0.32857143 -0.31428571 -0.3 -0.28571429 -0.27142857 -0.25714286 -0.24285714 -0.22857143 -0.21428571 -0.2 -0.18571429 -0.17142857 -0.15714286 -0.14285714 -0.12857143 -0.11428571 -0.1 -0.08571429 -0.07142857 -0.05714286 -0.04285714 -0.02857143 -0.01428571 0 0 0 0 0 0
  line L21 (-4.5955, -36.6696) -> (-4.6793, -36.6055)
  arc A43 (-4.7826, -35.9178) -> (-4.6793, -36.6055) centre (-4.3757, -36.2083) ccw
  arc A44 (-4.7826, -35.9178) -> (-4.5038, -35.5138) centre (-17.3506, -26.9445) ccw
  arc A45 (-3.8241, -35.3665) -> (-4.5038, -35.5138) centre (-4.0878, -35.7913) ccw
  line L22 (-3.8241, -35.3665) -> (-3.7345, -35.4221)
  spline S22 degree 5 poles (-3.7345, -35.4221) (-3.7287, -35.4257) (-3.717, -35.4328) (-3.6992, -35.443) (-3.675, -35.4557) (-3.6442, -35.4705) (-3.6128, -35.4845) (-3.5812, -35.498) (-3.5495, -35.5112) (-3.5176, -35.5242) (-3.4856, -35.537) (-3.4534, -35.5496) (-3.4211, -35.5618) (-3.3885, -35.5736) (-3.3558, -35.5851) (-3.3228, -35.5961) (-3.2897, -35.6069) (-3.2564, -35.6173) (-3.223, -35.6275) (-3.1895, -35.6375) (-3.1559, -35.6473) (-3.1222, -35.6568) (-3.0883, -35.6661) (-3.0543, -35.6752) (-3.0202, -35.684) (-2.986, -35.6925) (-2.9517, -35.7008) (-2.9172, -35.7089) (-2.8827, -35.7168) (-2.848, -35.7245) (-2.8133, -35.7319) (-2.7784, -35.7392) (-2.7435, -35.7462) (-2.7085, -35.753) (-2.6734, -35.7597) (-2.6382, -35.7661) (-2.6029, -35.7723) (-2.5675, -35.7783) (-2.532, -35.7842) (-2.4964, -35.7898) (-2.4608, -35.7953) (-2.4251, -35.8006) (-2.3893, -35.8056) (-2.3534, -35.8105) (-2.3175, -35.8152) (-2.2815, -35.8198) (-2.2454, -35.8241) (-2.2092, -35.8283) (-2.173, -35.8322) (-2.1367, -35.836) (-2.1003, -35.8397) (-2.0639, -35.8431) (-2.0274, -35.8464) (-1.9908, -35.8495) (-1.9542, -35.8524) (-1.9174, -35.8552) (-1.8807, -35.8578) (-1.8439, -35.8602) (-1.807, -35.8625) (-1.77, -35.8645) (-1.733, -35.8665) (-1.696, -35.8682) (-1.6588, -35.8698) (-1.6217, -35.8712) (-1.5844, -35.8725) (-1.5472, -35.8736) (-1.5098, -35.8745) (-1.4724, -35.8753) (-1.435, -35.8759) (-1.3975, -35.8763) (-1.3599, -35.8766) (-1.3299, -35.8767) (-1.3073, -35.8767) (-1.2922, -35.8767) (-1.2847, -35.8767) knots 0 0 0 0 0 0 0.01428571 0.02857143 0.04285714 0.05714286 0.07142857 0.08571429 0.1 0.11428571 0.12857143 0.14285714 0.15714286 0.17142857 0.18571429 0.2 0.21428571 0.22857143 0.24285714 0.25714286 0.27142857 0.28571429 0.3 0.31428571 0.32857143 0.34285714 0.35714286 0.37142857 0.38571429 0.4 0.41428571 0.42857143 0.44285714 0.45714286 0.47142857 0.48571429 0.5 0.51428571 0.52857143 0.54285714 0.55714286 0.57142857 0.58571429 0.6 0.61428571 0.62857143 0.64285714 0.65714286 0.67142857 0.68571429 0.7 0.71428571 0.72857143 0.74285714 0.75714286 0.77142857 0.78571429 0.8 0.81428571 0.82857143 0.84285714 0.85714286 0.87142857 0.88571429 0.9 0.91428571 0.92857143 0.94285714 0.95714286 0.97142857 0.98571429 1 1 1 1 1 1
  arc A46 (-1.2847, -35.8767) -> (-0.8731, -35.0924) centre (-17.3506, -26.9445) ccw
  spline S23 degree 5 poles (-0.8731, -35.0924) (-0.8774, -35.0862) (-0.8859, -35.0738) (-0.8987, -35.0552) (-0.9159, -35.0305) (-0.9375, -34.9998) (-0.9591, -34.9692) (-0.9809, -34.9387) (-1.0028, -34.9084) (-1.0247, -34.8782) (-1.0468, -34.8481) (-1.069, -34.8182) (-1.0913, -34.7884) (-1.1137, -34.7588) (-1.1362, -34.7293) (-1.1588, -34.6999) (-1.1815, -34.6707) (-1.2043, -34.6416) (-1.2272, -34.6127) (-1.2502, -34.5839) (-1.2733, -34.5552) (-1.2966, -34.5268) (-1.3199, -34.4984) (-1.3433, -34.4702) (-1.3669, -34.4422) (-1.3905, -34.4143) (-1.4143, -34.3866) (-1.4381, -34.3591) (-1.4621, -34.3317) (-1.4862, -34.3044) (-1.5104, -34.2773) (-1.5347, -34.2504) (-1.5591, -34.2237) (-1.5836, -34.1971) (-1.6082, -34.1707) (-1.6329, -34.1445) (-1.6578, -34.1185) (-1.6827, -34.0926) (-1.7078, -34.0669) (-1.7329, -34.0414) (-1.7582, -34.016) (-1.7836, -33.9909) (-1.8092, -33.966) (-1.8348, -33.9412) (-1.8606, -33.9167) (-1.8864, -33.8923) (-1.9124, -33.8681) (-1.9385, -33.8442) (-1.9648, -33.8204) (-1.9911, -33.7969) (-2.0176, -33.7736) (-2.0442, -33.7505) (-2.0709, -33.7277) (-2.0978, -33.7051) (-2.1248, -33.6827) (-2.152, -33.6606) (-2.1792, -33.6387) (-2.2066, -33.617) (-2.2341, -33.5956) (-2.2618, -33.5744) (-2.2896, -33.5536) (-2.3176, -33.5331) (-2.3458, -33.5131) (-2.3742, -33.4934) (-2.4028, -33.4741) (-2.4316, -33.455) (-2.4604, -33.4362) (-2.4893, -33.4175) (-2.5184, -33.3992) (-2.5477, -33.3813) (-2.5774, -33.3644) (-2.6016, -33.3517) (-2.6201, -33.3428) (-2.6326, -33.3372) (-2.6388, -33.3345) knots -1 -1 -1 -1 -1 -1 -0.98571429 -0.97142857 -0.95714286 -0.94285714 -0.92857143 -0.91428571 -0.9 -0.88571429 -0.87142857 -0.85714286 -0.84285714 -0.82857143 -0.81428571 -0.8 -0.78571429 -0.77142857 -0.75714286 -0.74285714 -0.72857143 -0.71428571 -0.7 -0.68571429 -0.67142857 -0.65714286 -0.64285714 -0.62857143 -0.61428571 -0.6 -0.58571429 -0.57142857 -0.55714286 -0.54285714 -0.52857143 -0.51428571 -0.5 -0.48571429 -0.47142857 -0.45714286 -0.44285714 -0.42857143 -0.41428571 -0.4 -0.38571429 -0.37142857 -0.35714286 -0.34285714 -0.32857143 -0.31428571 -0.3 -0.28571429 -0.27142857 -0.25714286 -0.24285714 -0.22857143 -0.21428571 -0.2 -0.18571429 -0.17142857 -0.15714286 -0.14285714 -0.12857143 -0.11428571 -0.1 -0.08571429 -0.07142857 -0.05714286 -0.04285714 -0.02857143 -0.01428571 0 0 0 0 0 0
  line L23 (-2.6388, -33.3345) -> (-2.7355, -33.2924)
  arc A47 (-3.0004, -32.6493) -> (-2.7355, -33.2924) centre (-2.5358, -32.834) ccw
  arc A48 (-3.0004, -32.6493) -> (-2.8263, -32.1904) centre (-17.3506, -26.9445) ccw
  arc A49 (-2.2016, -31.8847) -> (-2.8263, -32.1904) centre (-2.3561, -32.3602) ccw
  line L24 (-2.2016, -31.8847) -> (-2.1013, -31.9172)
  spline S24 degree 5 poles (-2.1013, -31.9172) (-2.0948, -31.9193) (-2.0818, -31.9234) (-2.0621, -31.929) (-2.0355, -31.9356) (-2.002, -31.9426) (-1.9683, -31.9487) (-1.9344, -31.9542) (-1.9004, -31.9594) (-1.8663, -31.9644) (-1.8321, -31.9692) (-1.7979, -31.9737) (-1.7636, -31.9779) (-1.7292, -31.9816) (-1.6946, -31.9848) (-1.66, -31.9877) (-1.6252, -31.9902) (-1.5904, -31.9923) (-1.5556, -31.9943) (-1.5207, -31.996) (-1.4857, -31.9974) (-1.4506, -31.9986) (-1.4155, -31.9995) (-1.3804, -32.0002) (-1.3452, -32.0005) (-1.3099, -32.0006) (-1.2745, -32.0005) (-1.2392, -32.0001) (-1.2037, -31.9995) (-1.1683, -31.9986) (-1.1327, -31.9976) (-1.0972, -31.9963) (-1.0616, -31.9947) (-1.0259, -31.993) (-0.9903, -31.991) (-0.9545, -31.9888) (-0.9188, -31.9864) (-0.883, -31.9838) (-0.8471, -31.981) (-0.8113, -31.978) (-0.7754, -31.9747) (-0.7394, -31.9713) (-0.7035, -31.9677) (-0.6675, -31.9638) (-0.6314, -31.9598) (-0.5954, -31.9556) (-0.5593, -31.9512) (-0.5232, -31.9465) (-0.487, -31.9417) (-0.4509, -31.9367) (-0.4147, -31.9316) (-0.3785, -31.9262) (-0.3423, -31.9206) (-0.306, -31.9149) (-0.2697, -31.909) (-0.2334, -31.9029) (-0.1971, -31.8966) (-0.1608, -31.8901) (-0.1244, -31.8835) (-0.0881, -31.8767) (-0.0517, -31.8697) (-0.0153, -31.8625) (0.0211, -31.8552) (0.0576, -31.8476) (0.094, -31.8399) (0.1305, -31.8321) (0.167, -31.824) (0.2035, -31.8158) (0.24, -31.8075) (0.2765, -31.7989) (0.313, -31.7902) (0.3422, -31.7831) (0.3641, -31.7777) (0.3788, -31.7741) (0.3861, -31.7723) knots 0 0 0 0 0 0 0.01428571 0.02857143 0.04285714 0.05714286 0.07142857 0.08571429 0.1 0.11428571 0.12857143 0.14285714 0.15714286 0.17142857 0.18571429 0.2 0.21428571 0.22857143 0.24285714 0.25714286 0.27142857 0.28571429 0.3 0.31428571 0.32857143 0.34285714 0.35714286 0.37142857 0.38571429 0.4 0.41428571 0.42857143 0.44285714 0.45714286 0.47142857 0.48571429 0.5 0.51428571 0.52857143 0.54285714 0.55714286 0.57142857 0.58571429 0.6 0.61428571 0.62857143 0.64285714 0.65714286 0.67142857 0.68571429 0.7 0.71428571 0.72857143 0.74285714 0.75714286 0.77142857 0.78571429 0.8 0.81428571 0.82857143 0.84285714 0.85714286 0.87142857 0.88571429 0.9 0.91428571 0.92857143 0.94285714 0.95714286 0.97142857 0.98571429 1 1 1 1 1 1
  arc A50 (0.3861, -31.7723) -> (0.598, -30.9124) centre (-17.3506, -26.9445) ccw
  spline S25 degree 5 poles (0.598, -30.9124) (0.5924, -30.9073) (0.5811, -30.8973) (0.5642, -30.8824) (0.5417, -30.8625) (0.5134, -30.8378) (0.485, -30.8133) (0.4566, -30.7889) (0.4281, -30.7647) (0.3995, -30.7406) (0.3709, -30.7167) (0.3422, -30.693) (0.3134, -30.6694) (0.2846, -30.6459) (0.2557, -30.6227) (0.2267, -30.5996) (0.1977, -30.5766) (0.1686, -30.5539) (0.1394, -30.5313) (0.1102, -30.5088) (0.0809, -30.4865) (0.0515, -30.4644) (0.0221, -30.4425) (-0.0074, -30.4208) (-0.037, -30.3992) (-0.0666, -30.3778) (-0.0963, -30.3565) (-0.1261, -30.3355) (-0.1559, -30.3146) (-0.1858, -30.2939) (-0.2158, -30.2734) (-0.2458, -30.2531) (-0.2759, -30.233) (-0.3061, -30.2131) (-0.3363, -30.1933) (-0.3666, -30.1738) (-0.3969, -30.1544) (-0.4273, -30.1353) (-0.4578, -30.1163) (-0.4884, -30.0976) (-0.519, -30.0791) (-0.5497, -30.0607) (-0.5804, -30.0426) (-0.6112, -30.0247) (-0.6421, -30.007) (-0.6731, -29.9896) (-0.7041, -29.9724) (-0.7352, -29.9553) (-0.7663, -29.9386) (-0.7975, -29.922) (-0.8288, -29.9057) (-0.8602, -29.8897) (-0.8916, -29.8739) (-0.9231, -29.8584) (-0.9547, -29.8432) (-0.9863, -29.8282) (-1.018, -29.8135) (-1.0498, -29.799) (-1.0817, -29.7847) (-1.1136, -29.7708) (-1.1456, -29.7572) (-1.1777, -29.744) (-1.2099, -29.7313) (-1.2422, -29.719) (-1.2746, -29.7071) (-1.307, -29.6955) (-1.3395, -29.6841) (-1.3721, -29.6729) (-1.4047, -29.662) (-1.4374, -29.6517) (-1.4703, -29.6423) (-1.4968, -29.6358) (-1.5169, -29.6317) (-1.5303, -29.6292) (-1.5371, -29.6281) knots -1 -1 -1 -1 -1 -1 -0.98571429 -0.97142857 -0.95714286 -0.94285714 -0.92857143 -0.91428571 -0.9 -0.88571429 -0.87142857 -0.85714286 -0.84285714 -0.82857143 -0.81428571 -0.8 -0.78571429 -0.77142857 -0.75714286 -0.74285714 -0.72857143 -0.71428571 -0.7 -0.68571429 -0.67142857 -0.65714286 -0.64285714 -0.62857143 -0.61428571 -0.6 -0.58571429 -0.57142857 -0.55714286 -0.54285714 -0.52857143 -0.51428571 -0.5 -0.48571429 -0.47142857 -0.45714286 -0.44285714 -0.42857143 -0.41428571 -0.4 -0.38571429 -0.37142857 -0.35714286 -0.34285714 -0.32857143 -0.31428571 -0.3 -0.28571429 -0.27142857 -0.25714286 -0.24285714 -0.22857143 -0.21428571 -0.2 -0.18571429 -0.17142857 -0.15714286 -0.14285714 -0.12857143 -0.11428571 -0.1 -0.08571429 -0.07142857 -0.05714286 -0.04285714 -0.02857143 -0.01428571 0 0 0 0 0 0
  line L25 (-1.5371, -29.6281) -> (-1.641, -29.6103)
  arc A51 (-2.0521, -29.0493) -> (-1.641, -29.6103) centre (-1.5568, -29.1174) ccw
  arc A52 (-2.0521, -29.0493) -> (-1.993, -28.562) centre (-17.3506, -26.9445) ccw
  arc A53 (-1.4596, -28.1157) -> (-1.993, -28.562) centre (-1.4957, -28.6144) ccw
  line L26 (-1.4596, -28.1157) -> (-1.3544, -28.1233)
  spline S26 degree 5 poles (-1.3544, -28.1233) (-1.3476, -28.1238) (-1.3339, -28.1247) (-1.3134, -28.1254) (-1.2861, -28.1254) (-1.2519, -28.1242) (-1.2177, -28.1221) (-1.1834, -28.1193) (-1.1492, -28.1162) (-1.1149, -28.1129) (-1.0806, -28.1094) (-1.0463, -28.1056) (-1.012, -28.1014) (-0.9776, -28.0967) (-0.9433, -28.0916) (-0.909, -28.0861) (-0.8747, -28.0802) (-0.8404, -28.074) (-0.8061, -28.0675) (-0.7717, -28.0608) (-0.7374, -28.0538) (-0.7031, -28.0466) (-0.6688, -28.0391) (-0.6345, -28.0313) (-0.6003, -28.0233) (-0.566, -28.0149) (-0.5317, -28.0063) (-0.4974, -27.9975) (-0.4632, -27.9884) (-0.429, -27.9791) (-0.3947, -27.9695) (-0.3605, -27.9598) (-0.3263, -27.9498) (-0.2921, -27.9395) (-0.2579, -27.9291) (-0.2238, -27.9184) (-0.1896, -27.9075) (-0.1555, -27.8964) (-0.1214, -27.8851) (-0.0873, -27.8736) (-0.0532, -27.8618) (-0.0191, -27.8499) (0.0149, -27.8378) (0.049, -27.8254) (0.083, -27.8129) (0.117, -27.8002) (0.151, -27.7872) (0.1849, -27.7741) (0.2188, -27.7608) (0.2528, -27.7473) (0.2867, -27.7336) (0.3205, -27.7197) (0.3544, -27.7057) (0.3882, -27.6914) (0.422, -27.677) (0.4558, -27.6624) (0.4895, -27.6476) (0.5233, -27.6326) (0.557, -27.6175) (0.5907, -27.6021) (0.6243, -27.5866) (0.6579, -27.571) (0.6916, -27.5551) (0.7251, -27.5391) (0.7587, -27.5229) (0.7922, -27.5066) (0.8257, -27.49) (0.8592, -27.4733) (0.8926, -27.4565) (0.926, -27.4394) (0.9594, -27.4222) (0.9861, -27.4084) (1.0061, -27.3979) (1.0194, -27.3908) (1.026, -27.3873) knots 0 0 0 0 0 0 0.01428571 0.02857143 0.04285714 0.05714286 0.07142857 0.08571429 0.1 0.11428571 0.12857143 0.14285714 0.15714286 0.17142857 0.18571429 0.2 0.21428571 0.22857143 0.24285714 0.25714286 0.27142857 0.28571429 0.3 0.31428571 0.32857143 0.34285714 0.35714286 0.37142857 0.38571429 0.4 0.41428571 0.42857143 0.44285714 0.45714286 0.47142857 0.48571429 0.5 0.51428571 0.52857143 0.54285714 0.55714286 0.57142857 0.58571429 0.6 0.61428571 0.62857143 0.64285714 0.65714286 0.67142857 0.68571429 0.7 0.71428571 0.72857143 0.74285714 0.75714286 0.77142857 0.78571429 0.8 0.81428571 0.82857143 0.84285714 0.85714286 0.87142857 0.88571429 0.9 0.91428571 0.92857143 0.94285714 0.95714286 0.97142857 0.98571429 1 1 1 1 1 1
  arc A54 (1.026, -27.3873) -> (1.026, -26.5017) centre (-17.3506, -26.9445) ccw
  spline S27 degree 5 poles (1.026, -26.5017) (1.0194, -26.4981) (1.0061, -26.4911) (0.9861, -26.4806) (0.9594, -26.4667) (0.926, -26.4495) (0.8926, -26.4325) (0.8592, -26.4157) (0.8257, -26.399) (0.7922, -26.3824) (0.7587, -26.3661) (0.7251, -26.3499) (0.6916, -26.3339) (0.6579, -26.318) (0.6243, -26.3023) (0.5907, -26.2868) (0.557, -26.2715) (0.5233, -26.2564) (0.4895, -26.2414) (0.4558, -26.2266) (0.422, -26.212) (0.3882, -26.1976) (0.3544, -26.1833) (0.3205, -26.1692) (0.2867, -26.1554) (0.2528, -26.1417) (0.2188, -26.1282) (0.1849, -26.1149) (0.151, -26.1017) (0.117, -26.0888) (0.083, -26.0761) (0.049, -26.0635) (0.0149, -26.0512) (-0.0191, -26.0391) (-0.0532, -26.0271) (-0.0873, -26.0154) (-0.1214, -26.0039) (-0.1555, -25.9926) (-0.1896, -25.9815) (-0.2238, -25.9706) (-0.2579, -25.9599) (-0.2921, -25.9494) (-0.3263, -25.9392) (-0.3605, -25.9292) (-0.3947, -25.9194) (-0.429, -25.9099) (-0.4632, -25.9006) (-0.4974, -25.8915) (-0.5317, -25.8827) (-0.566, -25.8741) (-0.6003, -25.8657) (-0.6345, -25.8577) (-0.6688, -25.8499) (-0.7031, -25.8424) (-0.7374, -25.8351) (-0.7717, -25.8282) (-0.8061, -25.8214) (-0.8404, -25.815) (-0.8747, -25.8088) (-0.909, -25.8029) (-0.9433, -25.7974) (-0.9776, -25.7922) (-1.012, -25.7876) (-1.0463, -25.7834) (-1.0806, -25.7796) (-1.1149, -25.7761) (-1.1492, -25.7728) (-1.1834, -25.7697) (-1.2177, -25.7669) (-1.2519, -25.7648) (-1.2861, -25.7635) (-1.3134, -25.7636) (-1.3339, -25.7643) (-1.3476, -25.7652) (-1.3544, -25.7656) knots -1 -1 -1 -1 -1 -1 -0.98571429 -0.97142857 -0.95714286 -0.94285714 -0.92857143 -0.91428571 -0.9 -0.88571429 -0.87142857 -0.85714286 -0.84285714 -0.82857143 -0.81428571 -0.8 -0.78571429 -0.77142857 -0.75714286 -0.74285714 -0.72857143 -0.71428571 -0.7 -0.68571429 -0.67142857 -0.65714286 -0.64285714 -0.62857143 -0.61428571 -0.6 -0.58571429 -0.57142857 -0.55714286 -0.54285714 -0.52857143 -0.51428571 -0.5 -0.48571429 -0.47142857 -0.45714286 -0.44285714 -0.42857143 -0.41428571 -0.4 -0.38571429 -0.37142857 -0.35714286 -0.34285714 -0.32857143 -0.31428571 -0.3 -0.28571429 -0.27142857 -0.25714286 -0.24285714 -0.22857143 -0.21428571 -0.2 -0.18571429 -0.17142857 -0.15714286 -0.14285714 -0.12857143 -0.11428571 -0.1 -0.08571429 -0.07142857 -0.05714286 -0.04285714 -0.02857143 -0.01428571 0 0 0 0 0 0
  line L27 (-1.3544, -25.7656) -> (-1.4596, -25.7733)
  arc A55 (-1.993, -25.327) -> (-1.4596, -25.7733) centre (-1.4957, -25.2746) ccw
  arc A56 (-1.993, -25.327) -> (-2.0521, -24.8397) centre (-17.3506, -26.9445) ccw
  arc A57 (-1.641, -24.2787) -> (-2.0521, -24.8397) centre (-1.5568, -24.7715) ccw
  line L28 (-1.641, -24.2787) -> (-1.5371, -24.2609)
  spline S28 degree 5 poles (-1.5371, -24.2609) (-1.5303, -24.2598) (-1.5169, -24.2573) (-1.4968, -24.2531) (-1.4703, -24.2466) (-1.4374, -24.2373) (-1.4047, -24.227) (-1.3721, -24.2161) (-1.3395, -24.2049) (-1.307, -24.1935) (-1.2746, -24.1819) (-1.2422, -24.17) (-1.2099, -24.1577) (-1.1777, -24.1449) (-1.1456, -24.1318) (-1.1136, -24.1182) (-1.0817, -24.1043) (-1.0498, -24.09) (-1.018, -24.0755) (-0.9863, -24.0608) (-0.9547, -24.0458) (-0.9231, -24.0306) (-0.8916, -24.0151) (-0.8602, -23.9993) (-0.8288, -23.9833) (-0.7975, -23.967) (-0.7663, -23.9504) (-0.7352, -23.9336) (-0.7041, -23.9166) (-0.6731, -23.8994) (-0.6421, -23.8819) (-0.6112, -23.8643) (-0.5804, -23.8464) (-0.5497, -23.8283) (-0.519, -23.8099) (-0.4884, -23.7914) (-0.4578, -23.7726) (-0.4273, -23.7537) (-0.3969, -23.7345) (-0.3666, -23.7152) (-0.3363, -23.6956) (-0.3061, -23.6759) (-0.2759, -23.656) (-0.2458, -23.6358) (-0.2158, -23.6155) (-0.1858, -23.595) (-0.1559, -23.5744) (-0.1261, -23.5535) (-0.0963, -23.5324) (-0.0666, -23.5112) (-0.037, -23.4898) (-0.0074, -23.4682) (0.0221, -23.4465) (0.0515, -23.4245) (0.0809, -23.4024) (0.1102, -23.3802) (0.1394, -23.3577) (0.1686, -23.3351) (0.1977, -23.3123) (0.2267, -23.2894) (0.2557, -23.2663) (0.2846, -23.243) (0.3134, -23.2196) (0.3422, -23.196) (0.3709, -23.1723) (0.3995, -23.1484) (0.4281, -23.1243) (0.4566, -23.1001) (0.485, -23.0757) (0.5134, -23.0512) (0.5417, -23.0265) (0.5642, -23.0066) (0.5811, -22.9916) (0.5924, -22.9816) (0.598, -22.9766) knots 0 0 0 0 0 0 0.01428571 0.02857143 0.04285714 0.05714286 0.07142857 0.08571429 0.1 0.11428571 0.12857143 0.14285714 0.15714286 0.17142857 0.18571429 0.2 0.21428571 0.22857143 0.24285714 0.25714286 0.27142857 0.28571429 0.3 0.31428571 0.32857143 0.34285714 0.35714286 0.37142857 0.38571429 0.4 0.41428571 0.42857143 0.44285714 0.45714286 0.47142857 0.48571429 0.5 0.51428571 0.52857143 0.54285714 0.55714286 0.57142857 0.58571429 0.6 0.61428571 0.62857143 0.64285714 0.65714286 0.67142857 0.68571429 0.7 0.71428571 0.72857143 0.74285714 0.75714286 0.77142857 0.78571429 0.8 0.81428571 0.82857143 0.84285714 0.85714286 0.87142857 0.88571429 0.9 0.91428571 0.92857143 0.94285714 0.95714286 0.97142857 0.98571429 1 1 1 1 1 1
  arc A58 (0.598, -22.9766) -> (0.3861, -22.1167) centre (-17.3506, -26.9445) ccw